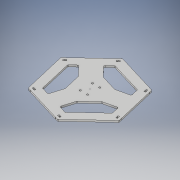
# Autodesk Inventor part: Hex_Servo_Top
Saved by Autodesk Inventor 2019 (Build 230136000, 136)
## iProperties
Created: 2019-09-26
Part Number: Hex_Servo_Top
Material: Generic
Document SubType Name: Modeling
Designer: Jorian Bruslind
Density: 1 g/cm^3
Appearance: Default
Author: Jorian Bruslind
Autodesk Inventor part; units mm, degrees
ref_plane "YZ Plane" through (0, 0, 0) normal (1, 0, 0) x (0, 1, 0)
ref_plane "XZ Plane" through (0, 0, 0) normal (0, 1, 0) x (-1, 0, 0)
ref_plane "XY Plane" through (0, 0, 0) normal (0, 0, 1) x (1, 0, 0)
sketch "Sketch1" plane through (0, 0, 0) normal (0, 1, 0) x (-1, 0, 0)
  line L0 (54.6535, 51.3614) -> (71.807, -21.6506)
  line L1 (71.807, -21.6506) -> (17.1535, -73.012)
  line L2 (17.1535, -73.012) -> (-54.6535, -51.3614)
  line L3 (-54.6535, -51.3614) -> (-71.807, 21.6506)
  line L4 (-71.807, 21.6506) -> (-17.1535, 73.012)
  line L5 (-17.1535, 73.012) -> (54.6535, 51.3614)
  point P0 (0, 0)
  point P1 (0, 0)
  dimension "d0" = 75
  dimension "d17" = 21.6506
  constraints: 12 end point, 1 coincident, 13 other
  measures "d0" distance of L0.end L1.end
  measures "d17" vertical distance of L4.end L0.start
extrude "Extrusion1" add sketch "Sketch1" along normal blind 3
sketch "Sketch2" plane through (54.6535, 0, -51.3614) normal (0.9734938, 0, -0.2287136) x (-0.2287136, 0, -0.9734938)
  line L0 (0, 0) -> (0, 3) projected
  line L1 (0, 1.5) -> (-5, 1.5)
  line L2 (-75, 0) -> (-75, 3) projected
  line L3 (-75, 1.5) -> (-70, 1.5)
  circle A0 centre (-70, 1.5) radius 1
  circle A1 centre (-5, 1.5) radius 1
  point P0 (-37.5, 0)
  dimension "d4" = 5
  dimension "d5" = 5
  dimension "d6" = 2
  dimension "d7" = 2
  constraints: 4 end point, 2 centre point, 2 coincident, 2 horizontal, 2 midpoint
  measures "d4" distance of L1.start L1.end
  measures "d5" distance of L3.start L3.end
  measures "d6" diameter of A0
  measures "d7" diameter of A1
extrude "Extrusion2" cut sketch "Sketch2" against normal blind 10
sketch "Sketch3" plane through (0, 3, 0) normal (0, 1, 0) x (1, 0, 0)
  circle A0 centre (0, 0) radius 0.5
  dimension "d10" = 1
  constraints: 1 centre point, 1 coincident
  measures "d10" diameter of A0
extrude "Extrusion3" cut sketch "Sketch3" against normal blind 5
pattern_circular "Circular Pattern1" count 3 over 360 about axis through (0, 3, 0) along (0, -1, 0) of "Extrusion2"
sketch "Sketch4" plane through (0, 3, 0) normal (0, 1, 0) x (1, 0, 0)
  line L0 (0, 0) -> (0, 10.5)
  line L1 (0, 10.5) -> (-6.25, 10.5)
  circle A0 centre (-6.25, 10.5) radius 1.5
  circle A1 centre (6.25, 10.5) radius 1.5
  circle A2 centre (-6.25, -10.5) radius 1.5
  circle A3 centre (6.25, -10.5) radius 1.5
  dimension "d18" = 10.5
  dimension "d19" = 6.25
  dimension "d20" = 3
  dimension "d23" = 12.5
  dimension "d26" = 21
  constraints: 4 centre point, 4 end point, 2 vertical, 1 coincident, 1 horizontal, 1 perpendicular, 6 other
  measures "d18" distance of L0.start L0.end
  measures "d19" distance of L0.end L1.end
  measures "d20" diameter of A0
  measures "d23" distance of A0.centre A1.centre
  measures "d26" distance of A0.centre A2.centre
extrude "Extrusion4" cut sketch "Sketch4" against normal blind 5
sketch "Sketch5" plane through (0, 3, 0) normal (0, 1, 0) x (1, 0, 0)
  line L0 (-54.6535, -51.3614) -> (17.1535, -73.012) projected
  line L1 (17.1535, -73.012) -> (12.3664, -71.5687)
  line L2 (12.3664, -71.5687) -> (13.5211, -67.7389)
  line L3 (13.5211, -67.7389) -> (11.1275, -67.0173)
  line L4 (13.5211, -67.7389) -> (15.9146, -68.4606)
  line L5 (11.1275, -67.0173) -> (11.8492, -64.6237)
  line L6 (11.8492, -64.6237) -> (16.6363, -66.0671)
  line L7 (16.6363, -66.0671) -> (15.9146, -68.4606)
  point P0 (0, 0)
  dimension "d31" = 5
  dimension "d32" = 4
  dimension "d33" = 2.5
  dimension "d34" = 90
  dimension "d35" = 2.5
  dimension "d36" = 90
  dimension "d37" = 2.5
  dimension "d38" = 90
  dimension "d39" = 90
  constraints: 14 end point, 2 perpendicular, 1 point on line
  measures "d31" distance of L0.end L1.end
  measures "d32" distance of L1.end L2.end
  measures "d33" distance of L2.end L3.end
  measures "d34" angle of L3 L2
  measures "d35" distance of L2.end L4.end
  measures "d36" angle of L2 L4
  measures "d37" distance of L3.end L5.end
  measures "d38" angle of L3 L5
  measures "d39" angle of L5 L6
extrude "Extrusion5" cut sketch "Sketch5" against normal blind 5
pattern_linear "Rectangular Pattern1" count 2 spacing 65 along (-0.9574271, 0, -0.2886751) of "Extrusion5"
pattern_circular "Circular Pattern2" count 3 over 360 about axis through (0, 3, 0) along (0, -1, 0) of "Extrusion5", "Rectangular Pattern1"
sketch "Sketch6" plane through (0, 3, 0) normal (0, 1, 0) x (1, 0, 0)
  line L0 (-71.807, 21.6506) -> (-17.1535, 73.012) projected
  line L1 (-71.807, 21.6506) -> (-17.1535, 73.012)
  line L2 (-17.1535, 73.012) -> (54.6535, 51.3614) projected
  line L3 (-17.1535, 73.012) -> (54.6535, 51.3614)
  line L4 (54.6535, 51.3614) -> (71.807, -21.6506) projected
  line L5 (54.6535, 51.3614) -> (71.807, -21.6506)
  line L6 (71.807, -21.6506) -> (17.1535, -73.012) projected
  line L7 (71.807, -21.6506) -> (17.1535, -73.012)
  line L8 (17.1535, -73.012) -> (-54.6535, -51.3614)
  line L9 (-48.909, -53.0934) -> (-50.8238, -52.5161) projected
  line L10 (-54.6535, -51.3614) -> (-71.807, 21.6506)
  line L11 (-55.2239, 16.6506) -> (-13.1921, 56.1506)
  line L12 (-13.1921, 56.1506) -> (42.0318, 39.5)
  line L13 (42.0318, 39.5) -> (55.2239, -16.6506)
  line L14 (55.2239, -16.6506) -> (13.1921, -56.1506)
  line L15 (13.1921, -56.1506) -> (-42.0318, -39.5)
  line L16 (-42.0318, -39.5) -> (-55.2239, 16.6506)
  circle A0 centre (0, 0) radius 0.5 projected
  line L17 (0, 0) -> (6.8607, -29.205)
  line L18 (0, 0) -> (30, 0) construction
  line L19 (6.8613, -29.2044) -> (28.7224, -8.6601)
  line L20 (28.7224, -8.6601) -> (21.8611, 20.5443)
  line L21 (21.8611, 20.5443) -> (-6.8613, 29.2044)
  line L22 (-6.8613, 29.2044) -> (-28.7224, 8.6601)
  line L23 (-28.7224, 8.6601) -> (-21.8611, -20.5443)
  line L24 (-21.8611, -20.5443) -> (6.8613, -29.2044)
  line L25 (28.7224, -8.6601) -> (21.8611, 20.5443)
  line L26 (21.8611, 20.5443) -> (45.1972, 26.0269)
  line L27 (45.1972, 26.0269) -> (52.0585, -3.1775)
  line L28 (52.0585, -3.1775) -> (28.7224, -8.6601)
  line L29 (-6.8613, 29.2044) -> (-28.7224, 8.6601)
  line L30 (-28.7224, 8.6601) -> (-45.1386, 26.1285)
  line L31 (-45.1386, 26.1285) -> (-23.2774, 46.6728)
  line L32 (-23.2774, 46.6728) -> (-6.8613, 29.2044)
  line L33 (-21.8611, -20.5443) -> (6.8613, -29.2044)
  line L34 (6.8613, -29.2044) -> (-0.0587, -52.1554)
  line L35 (-0.0587, -52.1554) -> (-28.7811, -43.4952)
  line L36 (-28.7811, -43.4952) -> (-21.8611, -20.5443)
  dimension "d50" = 15
  dimension "d51" = 30
  dimension "d52" = 76.78
  dimension "d53" = 28.7224
  constraints: 64 end point, 9 parallel, 8 collinear, 3 perpendicular, 1 equal length, 1 horizontal, 10 other
  measures "d50" distance between parallel lines of L10 L16
  measures "d51" distance of L17.start L17.end
  measures "d52" angle of L17 L18
  measures "d53" horizontal distance of L20.end L21.end
extrude "Extrusion6" cut sketch "Sketch6" against normal blind 5 contours L11 L30 L23 L36 L15 L16 | L11 L12 L13 L26 L21 L32 | L34 L19 L28 L13 L14 L15
fillet "Fillet1" radius 2 18 edges at (52.0585, 1.5, 3.1775) (55.2239, 1.5, 16.6506) (13.1921, 1.5, 56.1506) (-0.0587, 1.5, 52.1554) (6.8613, 1.5, 29.2044) (28.7224, 1.5, 8.6601) (-13.1921, 1.5, -56.1506) (-23.2774, 1.5, -46.6728) (-6.8613, 1.5, -29.2044) (21.8611, 1.5, -20.5443) (45.1972, 1.5, -26.0269) (42.0318, 1.5, -39.5) (-28.7224, 1.5, -8.6601) (-21.8611, 1.5, 20.5443) (-45.1386, 1.5, -26.1285) (-55.2239, 1.5, -16.6506) (-42.0318, 1.5, 39.5) (-28.7811, 1.5, 43.4952)
fillet "Fillet2" radius 2 6 edges at (-71.807, 1.5, -21.6506) (-54.6535, 1.5, 51.3614) (17.1535, 1.5, 73.012) (71.807, 1.5, 21.6506) (54.6535, 1.5, -51.3614) (-17.1535, 1.5, -73.012)
body "Solid1"
